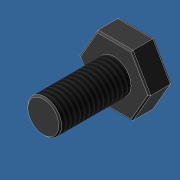
# Autodesk Inventor part: Small Bolt
Saved by Autodesk Inventor 2018 (Build 220112000, 112)
## iProperties
Created: 2018-04-08
Part Number: Small Bolt
Material: Generic
Document SubType Name: Modeling
Designer: Cole
Density: 1 g/cm^3
Appearance: Default
Author: Cole
Autodesk Inventor part; units mm, degrees
ref_plane "YZ Plane" through (0, 0, 0) normal (1, 0, 0) x (0, 1, 0)
ref_plane "XZ Plane" through (0, 0, 0) normal (0, 1, 0) x (-1, 0, 0)
ref_plane "XY Plane" through (0, 0, 0) normal (0, 0, 1) x (1, 0, 0)
sketch "Sketch1" plane through (0, 0, 0) normal (0, 0, 1) x (1, 0, 0)
  line L0 (7.9375, 0) -> (3.9688, -6.8741)
  line L1 (3.9688, -6.8741) -> (-3.9687, -6.8741)
  line L2 (-3.9687, -6.8741) -> (-7.9375, 0)
  line L3 (-7.9375, 0) -> (-3.9688, 6.8741)
  line L4 (-3.9688, 6.8741) -> (3.9688, 6.8741)
  line L5 (3.9688, 6.8741) -> (7.9375, 0)
  point P0 (0, 0)
  point P1 (0, 0)
  dimension "d0" = 15.875
  constraints: 12 end point, 1 coincident, 13 other
  measures "d0" distance of L0.start L2.end
extrude "Extrusion1" add sketch "Sketch1" along normal blind 5.08
sketch "Sketch2" plane through (0, 0, 5.08) normal (0, 0, 1) x (1, 0, 0)
  circle A0 centre (0, 0) radius 3.81
  dimension "d3" = 7.62
  constraints: 1 centre point, 1 coincident
  measures "d3" diameter of A0
extrude "Extrusion2" add sketch "Sketch2" along normal blind 16.002
thread "Thread1" size "10-24 UNC" class "2A" standard "ANSI Unified Screw Threads" full length
chamfer "Chamfer1" distance 0.3175 angle 45 1 edges at (-3.81, 0, 21.082)
fillet "Fillet1" radius 0.3175 12 edges at (5.9531, 3.437, 5.08) (0, 6.8741, 5.08) (-5.9531, 3.437, 5.08) (-5.9531, -3.437, 5.08) (0, -6.8741, 5.08) (5.9531, -3.437, 5.08) (5.9531, -3.437, 0) (0, -6.8741, 0) (-5.9531, -3.437, 0) (-5.9531, 3.437, 0) (0, 6.8741, 0) (5.9531, 3.437, 0)
body "Solid1"
